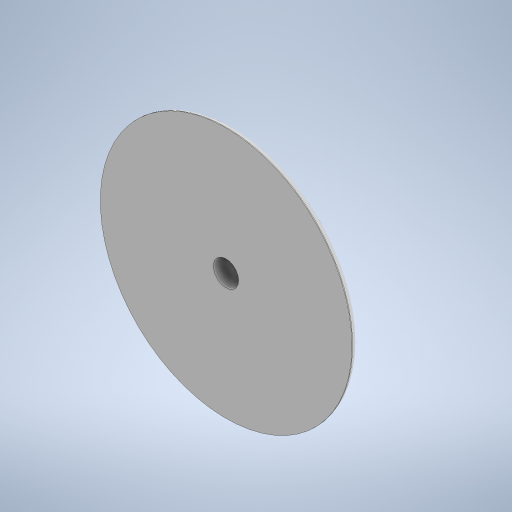
# Autodesk Inventor part: pritlacne_kolecko_polovina
Saved by Autodesk Inventor 2023.1 (Build 271208000, 208)
## iProperties
Created: 2023-01-11
Part Number: pritlacne_kolecko_polovina
Material: Generic
Document SubType Name: Modeling
Designer: zavrel
Density: 1 g/cm^3
Appearance: Default
Author: zavrel
Autodesk Inventor part; units mm, degrees
ref_plane "YZ Plane" through (0, 0, 0) normal (1, 0, 0) x (0, 1, 0)
ref_plane "XZ Plane" through (0, 0, 0) normal (0, 1, 0) x (-1, 0, 0)
sketch "Sketch1" plane through (0, 0, 0) normal (0, 1, 0) x (-1, 0, 0)
  line L0 (0, 0) -> (0, -5.5)
  line L1 (0, -5.5) -> (4.0342, -5.5)
  line L2 (4.0342, -5.5) -> (10, -3.15)
  line L3 (10, -3.15) -> (10, -2.35)
  line L4 (10, -2.35) -> (4.0342, 0)
  line L5 (4.0342, 0) -> (0, 0)
  point P0 (10, -2.75)
  dimension "d0" = 43
  dimension "d2" = 0.8
  dimension "d3" = 10
  dimension "d4" = 5.5
  constraints: 12 end point, 2 equal length, 1 horizontal, 1 midpoint, 1 parallel, 1 perpendicular, 1 vertical
  measures "d0" angle of L2 L4
  measures "d2" distance of L2.end L3.end
  measures "d3" distance from line of L0 point (10, -2.75)
  measures "d4" distance of L0.start L0.end
revolve "Revolution1" add sketch "Sketch1" angle 360 about axis through (0, 0, 0) along (0, 0, -1)
sketch "Sketch2" plane through (0, 0, -5.5) normal (0, 0, -1) x (-1, 0, 0)
  circle A0 centre (0, 0) radius 4.0342 projected
  circle A1 centre (0, 0) radius 1
  dimension "d6" = 2
  constraints: 1 centre point, 1 coincident
  measures "d6" diameter of A1
extrude "Extrusion1" cut sketch "Sketch2" against normal through all contours A1
ref_plane "Work Plane1" through (0, 0, -2.75) normal (0, 0, -1) x (-1, 0, 0)
fillet "Fillet1" radius 0.5 2 edges at (10, 0, -2.35) (10, 0, -3.15)
split "Split1" plane through (0, 0, -2.75) removes the side toward (0, 0, 1)
sketch "Sketch3" plane through (0, 0, -5.5) normal (0, 0, -1) x (-1, 0, 0)
  circle A0 centre (0, 0) radius 1 projected
  circle A1 centre (0, 0) radius 4.0342 projected
extrude "Extrusion2" add sketch "Sketch3" along normal blind 2
chamfer "Chamfer1" distance 0.5 angle 45 1 edges at (4.0342, 0, -7.5)
body "Solid1"
